baseplate v1 (Autodesk Fusion 360 design; units mm, degrees)
Autodesk Fusion 360 part; units mm, degrees
sketch "Sketch1" plane through (0, 0, 0) normal (0, 1, 0) x (1, 0, 0)
  line L0 (900, -200) -> (-900, -200)
  line L1 (-900, -200) -> (-900, 200)
  line L2 (-900, 200) -> (900, 200)
  line L3 (900, 200) -> (900, -200)
  line L4 (900, -200) -> (-900, 200) construction
  line L5 (-900, -200) -> (900, 200) construction
  dimension "d1" = 1800
  dimension "d2" = 400
  constraint horizontal L0
  constraint perpendicular L0 L1
  constraint parallel L0 L2
  constraint parallel L1 L3
  constraint coincident L4 origin
  constraint coincident L5 origin
  measures "d1" distance of L1.end L2.end
  measures "d2" distance of L0.end L1.end
extrude "Extrude1" add sketch "Sketch1" along normal blind 12
sketch "Sketch2" plane through (0, 12, 0) normal (0, 1, 0) x (-1, 0, 0)
  line L0 (-900, -200) -> (900, -200)
  line L1 (900, -200) -> (900, 200)
  line L2 (900, 200) -> (-900, 200)
  line L3 (-900, 200) -> (-900, -200)
  line L4 (0, 0) -> (900, 0)
  line L5 (900, 0) -> (875, 0)
  line L6 (875, 0) -> (875, -106)
  line L7 (875, -106) -> (102.85, -106)
  line L8 (102.85, -106) -> (102.85, 106)
  line L9 (102.85, 106) -> (875, 106)
  line L10 (875, 106) -> (875, -106)
  dimension "d5" = 25
  dimension "d6" = 106
  dimension "d7" = 772.15
  dimension "d8" = 212
  constraint coincident L4.start origin
  constraint midpoint L1 L4.end
  constraint perpendicular L1 L5
  constraint perpendicular L4 L6
  constraint horizontal L7
  constraint vertical L8
  constraint horizontal L9
  constraint vertical L10
  measures "d5" distance of L4.end L5.end
  measures "d6" distance of L5.end L6.end
  measures "d7" distance of L6.end L7.end
  measures "d8" distance of L6.end L9.end
hole "Hole1" at (-875, 12, -106) at (-102.85, 12, -106) at (-102.85, 12, 106) at (-875, 12, 106) direction (0, -1, 0) diameter 6.78 end through all
thread "Thread1" "ISO Metric profile 8.0 M8x1.25 6H" thread offset 0 thread depth 10
sketch "Sketch3" plane through (0, 12, 0) normal (0, 1, 0) x (-1, 0, 0)
  circle A0 centre (102.85, 106) radius 3.3898
  circle A1 centre (875, -106) radius 3.3898
  circle A2 centre (102.85, -106) radius 3.3898
  circle A3 centre (875, 106) radius 3.3898
  line L0 (-900, -200) -> (900, -200)
  line L1 (900, -200) -> (900, 200)
  line L2 (900, 200) -> (-900, 200)
  line L3 (-900, 200) -> (-900, -200)
equation "d6 = ( 212 / 2 ) * 1 mm"
